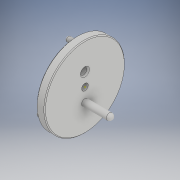
# Autodesk Inventor part: idk
Saved by Autodesk Inventor 2017 (Build 210142000, 142)
## iProperties
Created: 2017-04-17
Part Number: idk
Material: Generic
Document SubType Name: Modeling
Designer: 167942
Density: 1 g/cm^3
Appearance: Default
Author: 167942
Autodesk Inventor part; units mm, degrees
ref_plane "YZ Plane" through (0, 0, 0) normal (1, 0, 0) x (0, 1, 0)
ref_plane "XZ Plane" through (0, 0, 0) normal (0, 1, 0) x (-1, 0, 0)
ref_plane "XY Plane" through (0, 0, 0) normal (0, 0, 1) x (1, 0, 0)
sketch "Sketch1" plane through (0, 0, 0) normal (1, 0, 0) x (0, 1, 0)
  circle A0 centre (0, 0) radius 38.8938
  dimension "d0" = 77.7875
  constraints: 1 centre point, 1 coincident
  measures "d0" diameter of A0
extrude "Extrusion1" add sketch "Sketch1" along normal blind 7.9375
chamfer "Chamfer1" distance 0.7874 angle 45 2 edges at (7.9375, -38.8938, 0) (0, -38.8938, 0)
sketch "Sketch2" plane through (7.9375, 0, 0) normal (1, 0, 0) x (0, 0, -1)
  circle A0 centre (0, 0) radius 3.175
  dimension "d6" = 6.35
  constraints: 1 centre point, 1 coincident
  measures "d6" diameter of A0
extrude "Extrusion2" cut sketch "Sketch2" against normal blind 7.9375
sketch "Sketch3" plane through (0, 0, 0) normal (-1, 0, 0) x (0, 0, 1)
  line L0 (0, 0) -> (0, -12.7)
  dimension "d9" = 12.7
  constraints: 2 end point, 1 vertical
  measures "d9" distance of L0.start L0.end
hole "Hole1" at (0, -12.7, 0) direction (1, 0, 0) diameter 6.35 end through all countersink diameter 8.7376 countersink angle 82
sketch "Sketch4" plane through (0, 0, 0) normal (-1, 0, 0) x (0, 0, 1)
  point P0 (0, 0)
sketch "Sketch5" plane through (7.9375, 0, 0) normal (1, 0, 0) x (0, 0, -1)
  circle A0 centre (0, 0) radius 26.1938
  dimension "d17" = 52.3875
  constraints: 1 centre point, 1 coincident
  measures "d17" diameter of A0
extrude "Extrusion3" cut sketch "Sketch5" against normal blind 0.7874
sketch "Sketch6" plane through (0, 0, 0) normal (-1, 0, 0) x (0, 0, 1)
  line L0 (0, 0) -> (0, 12.7)
  circle A0 centre (0, 12.7) radius 3.175
  dimension "d20" = 12.7
  dimension "d21" = 6.35
  constraints: 2 end point, 1 centre point, 1 coincident, 1 vertical
  measures "d20" distance of L0.start L0.end
  measures "d21" diameter of A0
extrude "Extrusion4" add sketch "Sketch6" along normal blind 22.225
sketch "Sketch7" plane through (-22.225, 12.7, 0) normal (-1, 0, 0) x (0, 0, 1)
  circle A0 centre (0, 0) radius 3.175 projected
  circle A1 centre (0, 0) radius 3.175
  point P0 (0, -12.7)
  constraints: 1 centre point, 1 coincident
extrude "Extrusion5" add sketch "Sketch7" along normal blind 4.7625
fillet "Fillet1" radius 3.175 1 edges at (-26.9875, 12.7, -3.175)
sketch "Sketch8" plane through (7.9375, 0, 0) normal (1, 0, 0) x (0, 0, -1)
  circle A0 centre (0, -32.3239) radius 2.3813
  circle A1 centre (27.9933, 16.162) radius 2.3813
  circle A2 centre (-27.9933, 16.162) radius 2.3813
  point P0 (0, 0)
  dimension "d27" = 4.7625
  dimension "d30" = 360
  constraints: 3 centre point, 7 other
  measures "d27" diameter of A0
extrude "Extrusion6" add sketch "Sketch8" along normal blind 4.7625
sketch "Sketch9" plane through (12.7, 16.162, -27.9933) normal (1, 0, 0) x (0, 0, -1)
  circle A0 centre (0, 0) radius 2.3813
  point P0 (-27.9933, -16.162)
  constraints: 1 centre point
extrude "Extrusion7" add sketch "Sketch9" along normal blind 4.445
fillet "Fillet2" radius 1.5875 1 edges at (17.145, 16.162, -25.6121)
sketch "Sketch10" plane through (12.7, 16.162, 27.9933) normal (1, 0, 0) x (0, 0, -1)
  circle A0 centre (0, 0) radius 2.3813 projected
  circle A1 centre (0, 0) radius 2.3813
  point P0 (27.9933, -16.162)
  constraints: 1 centre point, 1 coincident
extrude "Extrusion8" add sketch "Sketch10" along normal blind 4.445
fillet "Fillet3" radius 1.5875 1 edges at (17.145, 16.162, 30.3746)
sketch "Sketch11" plane through (12.7, -32.3239, 0) normal (1, 0, 0) x (0, 0, -1)
  circle A0 centre (0, 0) radius 2.3813 projected
  circle A1 centre (0, 0) radius 2.3813
  point P0 (0, 32.3239)
  constraints: 1 centre point, 1 coincident
extrude "Extrusion9" add sketch "Sketch11" along normal blind 4.445
fillet "Fillet4" radius 1.5875 1 edges at (17.145, -32.3239, 2.3813)
body "Solid1"
